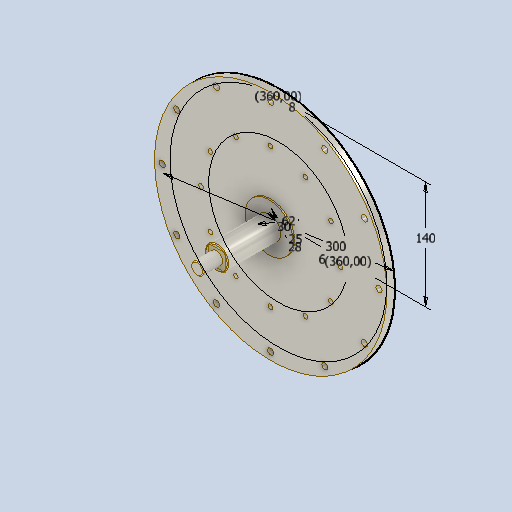
# Autodesk Inventor part: podstawa
Saved by Autodesk Inventor 2023 (Build 270158000, 158)
## iProperties
Created: 2023-03-26
Part Number: podstawa
Material: Tytan
Document SubType Name: Modeling
Designer: krzys
Density: 4.51 g/cm^3
Appearance: Tytan
Mass: 3411.79 g
Surface Area: 1621.57 cm^2
Volume: 756.494 cm^3
Author: krzys
## iProperties of the stored document podstawa_Drukowanie 3D.ipt
Created: 2023-04-25
Part Number: podstawa_Drukowanie 3D
Material: Ogólny
Document SubType Name: Modeling
Designer: krzys
Density: 1 g/cm^3
Appearance: Domyślna
Author: krzys
Autodesk Inventor part; units mm, degrees
ref_plane "YZ Plane" through (0, 0, 0) normal (1, 0, 0) x (0, 1, 0)
ref_plane "XZ Plane" through (0, 0, 0) normal (0, 1, 0) x (-1, 0, 0)
ref_plane "XY Plane" through (0, 0, 0) normal (0, 0, 1) x (1, 0, 0)
sketch "Szkic1" plane through (0, 0, 0) normal (0, 0, 1) x (1, 0, 0)
  circle A0 centre (0, 0) radius 150
  circle A1 centre (0, 0) radius 15
  circle A2 centre (0, 140) radius 4
  circle A3 centre (-70, 121.2436) radius 4
  circle A4 centre (-121.2436, 70) radius 4
  circle A5 centre (-140, 0) radius 4
  circle A6 centre (-121.2436, -70) radius 4
  circle A7 centre (-70, -121.2436) radius 4
  circle A8 centre (0, 0) radius 31
  circle A9 centre (0, -140) radius 4
  circle A10 centre (70, -121.2436) radius 4
  circle A11 centre (0, 0) radius 14
  circle A12 centre (0, 0) radius 12.5
  circle A13 centre (121.2436, -70) radius 4
  circle A14 centre (140, 0) radius 4
  circle A15 centre (121.2436, 70) radius 4
  circle A16 centre (70, 121.2436) radius 4
  circle A17 centre (90, 0) radius 3
  circle A18 centre (77.9423, 45) radius 3
  circle A19 centre (45, 77.9423) radius 3
  circle A20 centre (0, 90) radius 3
  circle A21 centre (-45, 77.9423) radius 3
  circle A22 centre (-77.9423, 45) radius 3
  circle A23 centre (-90, 0) radius 3
  circle A24 centre (-77.9423, -45) radius 3
  circle A25 centre (-45, -77.9423) radius 3
  circle A26 centre (0, -90) radius 3
  circle A27 centre (45, -77.9423) radius 3
  circle A28 centre (77.9423, -45) radius 3
  dimension "d0" = 300
  dimension "d1" = 30
  dimension "d2" = 8
  dimension "d5" = 360
  dimension "d7" = 62
  dimension "d8" = 140
  dimension "d15" = 28
  dimension "d16" = 25
  dimension "d31" = 6
  dimension "d34" = 360
  constraints: 29 centre point, 5 coincident, 50 other
  measures "d0" diameter of A0
  measures "d1" diameter of A1
  measures "d2" diameter of A2
  measures "d7" diameter of A8
  measures "d8" distance of A2.centre point (0, 0)
  measures "d15" diameter of A11
  measures "d16" diameter of A12
  measures "d31" diameter of A17
extrude "Wyciągnięcie proste1" add sketch "Szkic1" along normal blind 80 contours A1 | A11 | A12
extrude "Wyciągnięcie proste2" add sketch "Szkic1" along normal blind 12 contours A8
ref_plane "Płaszczyzna konstrukcyjna1" through (0, 0, 80) normal (0, 0, 1) x (1, 0, 0)
sketch "Szkic2" plane through (0, 0, 80) normal (0, 0, 1) x (1, 0, 0)
  circle A0 centre (0, 0) radius 8
  dimension "d21" = 16
  constraints: 1 centre point, 1 coincident
  measures "d21" diameter of A0
extrude "Wyciągnięcie proste6" add sketch "Szkic2" along normal blind 25
extrude "Wyciągnięcie proste8" add sketch "Szkic1" along normal blind 10 contours A0
chamfer "Faza2" distance 1 angle 45 1 edges at (-15, 0, 80)
thread "Gwint2" size "M16x2" class "6g" standard "ANSI Metric M Profile" full length
chamfer "Faza4" distance 1 angle 45 1 edges at (-8, 0, 105)
